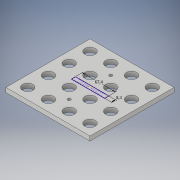
# Autodesk Inventor part: front_plate_2
Saved by Autodesk Inventor 2019 (Build 230136000, 136)
## iProperties
Created: 2019-08-25
Part Number: front_plate_2
Material: Generic
Document SubType Name: Modeling
Designer: Lino P
Density: 1 g/cm^3
Appearance: Default
Author: Lino P
Autodesk Inventor part; units mm, degrees
ref_plane "YZ Plane" through (0, 0, 0) normal (1, 0, 0) x (0, 1, 0)
ref_plane "XZ Plane" through (0, 0, 0) normal (0, 1, 0) x (-1, 0, 0)
ref_plane "XY Plane" through (0, 0, 0) normal (0, 0, 1) x (1, 0, 0)
sketch "Sketch1" plane through (0, 0, 0) normal (0, 1, 0) x (-1, 0, 0)
  line L0 (-85, 85) -> (85, 85)
  line L1 (85, 85) -> (85, -85)
  line L2 (85, -85) -> (-85, -85)
  line L3 (-85, -85) -> (-85, 85)
  line L4 (-85, 85) -> (85, -85) construction
  line L5 (85, 85) -> (-85, -85) construction
  point P0 (0, 0)
  point P1 (-63, -63)
  point P2 (-63, -21)
  point P3 (-63, 21)
  point P4 (-63, 63)
  point P5 (-21, -63)
  point P6 (-21, -21)
  point P7 (-21, 21)
  point P8 (-21, 63)
  point P9 (21, -63)
  point P10 (21, -21)
  point P11 (21, 21)
  point P12 (21, 63)
  point P13 (63, -63)
  point P14 (63, -21)
  point P15 (63, 21)
  point P16 (63, 63)
  dimension "d0" = 170
  dimension "d1" = 170
  dimension "d4" = 42
  dimension "d7" = 42
  constraints: 12 end point, 2 horizontal, 2 midpoint, 2 parallel, 1 perpendicular, 1 vertical, 15 other
  measures "d0" distance of L1.end L2.end
  measures "d1" distance of L0.end L1.end
  measures "d4" distance of point (-63, -63) point (-63, -21)
  measures "d7" distance of point (-63, -63) point (-21, -63)
extrude "Extrusion1" add sketch "Sketch1" along normal blind 9
hole "Hole1" at (63, 0, -63) at (63, 0, -21) at (63, 0, 21) at (63, 0, 63) at (21, 0, -63) at (21, 0, -21) at (21, 0, 21) at (21, 0, 63) at (-21, 0, -63) at (-21, 0, -21) at (-21, 0, 21) at (-21, 0, 63) at (-63, 0, -63) at (-63, 0, -21) at (-63, 0, 21) at (-63, 0, 63) direction (0, 1, 0) diameter 21 end through all both
sketch "Sketch2" plane through (0, 9, 0) normal (0, 1, 0) x (1, 0, 0)
  line L0 (-33.7, -4.15) -> (33.7, -4.15)
  line L1 (33.7, -4.15) -> (33.7, 4.15)
  line L2 (33.7, 4.15) -> (-33.7, 4.15)
  line L3 (-33.7, 4.15) -> (-33.7, -4.15)
  line L4 (-33.7, -4.15) -> (33.7, 4.15) construction
  line L5 (33.7, -4.15) -> (-33.7, 4.15) construction
  point P0 (0, 0)
  dimension "d19" = 67.4
  dimension "d20" = 8.3
  constraints: 12 end point, 2 midpoint, 2 parallel, 1 horizontal, 1 perpendicular
  measures "d19" distance of L2.end L1.end
  measures "d20" distance of L1.end L0.end
sketch "Sketch4" plane through (0, 9, 0) normal (0, 1, 0) x (1, 0, 0)
  line L0 (-85, 85) -> (85, 85) construction
  line L1 (-7.5, -85) -> (7.5, -85) construction
  line L2 (7.5, -85) -> (7.5, 85) construction
  line L3 (7.5, 85) -> (-7.5, 85) construction
  line L4 (-7.5, 85) -> (-7.5, -85) construction
  line L5 (-7.5, -85) -> (7.5, 85) construction
  line L6 (7.5, -85) -> (-7.5, 85) construction
  circle A0 centre (-63, -21) radius 10.5 construction
  circle A1 centre (-63, 63) radius 10.5 construction
  circle A2 centre (-21, -21) radius 10.5 construction
  circle A3 centre (-21, 63) radius 10.5 construction
  circle A4 centre (21, -21) radius 10.5 construction
  circle A5 centre (21, 63) radius 10.5 construction
  circle A6 centre (63, -21) radius 10.5 construction
  circle A7 centre (63, 63) radius 10.5 construction
  circle A8 centre (63, 21) radius 10.5 construction
  circle A9 centre (63, -63) radius 10.5 construction
  circle A10 centre (21, 21) radius 10.5 construction
  circle A11 centre (21, -63) radius 10.5 construction
  circle A12 centre (-21, 21) radius 10.5 construction
  circle A13 centre (-21, -63) radius 10.5 construction
  circle A14 centre (-63, 21) radius 10.5 construction
  circle A15 centre (-63, -63) radius 10.5 construction
  line L7 (-85, -85) -> (85, -85) construction
  line L8 (85, -85) -> (85, 85) construction
  line L9 (85, 85) -> (-85, 85) construction
  line L10 (-85, 85) -> (-85, -85) construction
  line L11 (-21, 63) -> (21, 63) construction
  line L12 (21, 63) -> (21, 21) construction
  line L13 (21, 21) -> (-21, 21) construction
  line L14 (-21, 21) -> (-21, 63) construction
  line L15 (-85, 0) -> (85, 0) construction
  point P0 (0, 0)
  point P1 (0, 42)
  point P2 (0, -42)
  dimension "d39" = 15
  constraints: 22 end point, 4 midpoint, 4 parallel, 2 horizontal, 2 perpendicular, 1 point on line, 1 symmetric about line
  measures "d39" distance of L3.end L2.end
hole "Hole4" at (0, 9, -42) at (0, 9, 42) direction (0, -1, 0) diameter 6 end through all both
body "Solid1"
